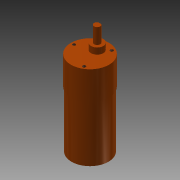
# Autodesk Inventor part: 知能ロボコンタミヤギヤードモータ540
Saved by Autodesk Inventor 2013 (Build 170138000, 138)
## iProperties
Created: 2014-06-18
Part Number: 知能ロボコンタミヤギヤードモータ540
Material: 鋼、炭素鋼
Document SubType Name: Modeling
Designer: horumo136
Density: 1 g/cm^3
Author: horumo136
Autodesk Inventor part; units mm, degrees
ref_plane "YZ Plane" through (0, 0, 0) normal (1, 0, 0) x (0, 1, 0)
ref_plane "XZ Plane" through (0, 0, 0) normal (0, 1, 0) x (-1, 0, 0)
ref_plane "XY Plane" through (0, 0, 0) normal (0, 0, 1) x (1, 0, 0)
sketch "スケッチ1" plane through (0, 0, 0) normal (0, 0, 1) x (1, 0, 0)
  circle A0 centre (0, 0) radius 17.9
  dimension "d0" = 35.8
  constraints: 1 centre point, 1 coincident
  measures "d0" diameter of A0
extrude "押し出し1" add sketch "スケッチ1" along normal blind 54.5
sketch "スケッチ2" plane through (0, 0, 54.5) normal (0, 0, 1) x (1, 0, 0)
  circle A0 centre (0, 0) radius 17.9 projected
  circle A1 centre (0, 0) radius 18.5
  dimension "d3" = 37
  constraints: 1 centre point, 1 coincident
  measures "d3" diameter of A1
extrude "押し出し2" add sketch "スケッチ2" along normal blind 27.5 contours A0 | A1
sketch "スケッチ3" plane through (0, 0, 82) normal (0, 0, 1) x (1, 0, 0)
  circle A0 centre (0, 0) radius 18.5 projected
  line L0 (0, 0) -> (0, 7)
  circle A1 centre (0, 7) radius 6
  dimension "d6" = 7
  dimension "d7" = 12
  constraints: 2 end point, 1 centre point, 1 coincident, 1 vertical
  measures "d6" distance of L0.start L0.end
  measures "d7" diameter of A1
extrude "押し出し3" add sketch "スケッチ3" along normal blind 6 contours A1
sketch "スケッチ4" plane through (0, 7, 88) normal (0, 0, 1) x (1, 0, 0)
  circle A0 centre (0, 0) radius 6 projected
  circle A1 centre (0, 0) radius 3
  point P0 (0, -7)
  dimension "d10" = 6
  constraints: 1 centre point, 1 coincident
  measures "d10" diameter of A1
extrude "押し出し4" add sketch "スケッチ4" along normal blind 15 contours A1
sketch "スケッチ5" plane through (0, 7, 103) normal (0, 0, 1) x (1, 0, 0)
  circle A0 centre (0, 0) radius 3 projected
  line L0 (0, -3) -> (0, 2.5)
  line L1 (0, 2.5) -> (1.6583, 2.5)
  line L2 (-1.6583, 2.5) -> (0, 2.5)
  point P0 (0, -7)
  dimension "d13" = 5.5
  constraints: 6 end point, 3 point on circle, 1 collinear, 1 perpendicular, 1 vertical
  measures "d13" distance of L0.start L0.end
extrude "押し出し5" cut sketch "スケッチ5" against normal blind 12 contours L1 L2 A0
sketch "スケッチ6" plane through (0, 0, 82) normal (0, 0, 1) x (1, 0, 0)
  circle A0 centre (0, 0) radius 18.5 projected
  circle A1 centre (0, 0) radius 15.5
  circle A2 centre (-15.5, 0) radius 1.5
  line L0 (0, 0) -> (7.75, 13.4234)
  line L1 (0, 0) -> (15.5, 0) construction
  line L2 (0, 0) -> (7.75, -13.4234)
  circle A3 centre (7.75, 13.4234) radius 1.5
  circle A4 centre (7.75, -13.4234) radius 1.5
  dimension "d16" = 31
  dimension "d17" = 3
  dimension "d18" = 60
  dimension "d19" = 3
  dimension "d20" = 3
  constraints: 6 end point, 4 centre point, 3 coincident, 3 point on circle, 1 equal length, 1 horizontal
  measures "d16" diameter of A1
  measures "d17" diameter of A2
  measures "d18" angle of L1 L0
  measures "d19" diameter of A3
  measures "d20" diameter of A4
hole "穴1" at (7.75, 13.4234, 82) at (-15.5, 0, 82) at (7.75, -13.4234, 82) direction (0, 0, -1) diameter 3 depth 3 tip angle 118
thread "ねじ1" size "M3x0.5" class "6H" standard "ANSI Metric M Profile" full length
thread "ねじ2" size "M3x0.5" class "6H" standard "ANSI Metric M Profile" full length
thread "ねじ3" size "M3x0.5" class "6H" standard "ANSI Metric M Profile" full length
